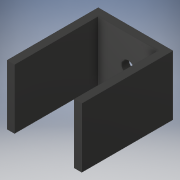
# Autodesk Inventor part: slotcar_beam
Saved by Autodesk Inventor 2019.4 (Build 234330000, 330)
## iProperties
Created: 2020-09-27
Part Number: slotcar_beam
Material: Generic
Document SubType Name: Modeling
Designer: deanv
Density: 1 g/cm^3
Appearance: Smooth - Black
Author: deanv
Autodesk Inventor part; units mm, degrees
ref_plane "YZ Plane" through (0, 0, 0) normal (1, 0, 0) x (0, 1, 0)
ref_plane "XZ Plane" through (0, 0, 0) normal (0, 1, 0) x (-1, 0, 0)
ref_plane "XY Plane" through (0, 0, 0) normal (0, 0, 1) x (1, 0, 0)
sketch "Sketch1" plane through (0, 0, 0) normal (0, 0, 1) x (1, 0, 0)
  line L0 (-12.5, -10) -> (12.5, -10)
  line L1 (12.5, -10) -> (12.5, 10)
  line L2 (12.5, 10) -> (-12.5, 10)
  line L3 (-12.5, 10) -> (-12.5, -10)
  line L4 (-12.5, -10) -> (12.5, 10) construction
  line L5 (12.5, -10) -> (-12.5, 10) construction
  line L6 (-12.5, 10) -> (-10, 10)
  line L7 (-10, 10) -> (-10, -10)
  line L8 (-10, -10) -> (-12.5, -10)
  line L9 (-12.5, -10) -> (-12.5, 10)
  line L10 (12.5, -10) -> (10, -10)
  line L11 (10, -10) -> (10, 10)
  line L12 (10, 10) -> (12.5, 10)
  line L13 (12.5, 10) -> (12.5, -10)
  point P0 (0, 0)
  point P1 (0, 0)
  dimension "d0" = 25
  dimension "d1" = 20
  dimension "d2" = 2.5
  dimension "d3" = 2.5
  constraints: 28 end point, 6 parallel, 3 horizontal, 3 perpendicular, 2 midpoint, 2 point on line, 1 coincident
  measures "d0" distance of L2.end L1.end
  measures "d1" distance of L1.end L0.end
  measures "d2" distance of L7.end L8.end
  measures "d3" distance of L11.end L12.end
extrude "Extrusion1" add sketch "Sketch1" along normal blind 2.5 contours L7 L2 L11 L0
extrude "Extrusion2" add sketch "Sketch1" along normal blind 30.5 contours L3 L2 L7 L0 | L11 L2 L1 L0
hole "Hole1" at (0, 0, 0) direction (0, 0, 1) diameter 4.5 end through all both
body "Solid1"
